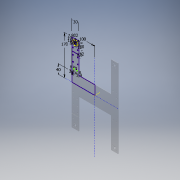
# Autodesk Inventor part: chassis mit motorlöcher
Saved by Autodesk Inventor 2018 (Build 220112000, 112)
## iProperties
Created: 2018-01-20
Part Number: chassis mit motorlöcher
Material: Polycarbonat, rauchfarben
Document SubType Name: Modeling
Designer: fhinstall
Density: 1.2 g/cm^3
Appearance: Polycarbonat - Rauch
Mass: 111.621 g
Surface Area: 687.489 cm^2
Volume: 93.0173 cm^3
Author: fhinstall
Autodesk Inventor part; units mm, degrees
ref_plane "YZ Plane" through (0, 0, 0) normal (1, 0, 0) x (0, 1, 0)
ref_plane "XZ Plane" through (0, 0, 0) normal (0, 1, 0) x (-1, 0, 0)
ref_plane "XY Plane" through (0, 0, 0) normal (0, 0, 1) x (1, 0, 0)
sketch "Skizze1" plane through (0, 0, 0) normal (0, 1, 0) x (-1, 0, 0)
  line L0 (127.3199, 0) -> (-102.7808, 0) construction
  line L1 (0, 142.2638) -> (0, -235.5235) construction
  line L2 (100, 50) -> (100, 0)
  line L3 (70, 40) -> (0, 40)
  line L4 (0, 0) -> (100, 0)
  line L5 (0, 40) -> (0, 0)
  line L6 (100, 50) -> (100, 170)
  line L7 (100, 170) -> (70, 170)
  line L8 (70, 170) -> (70, 40)
  circle A0 centre (95, 36) radius 1.7
  line L9 (100, 140) -> (70, 140) construction
  circle A1 centre (85, 155) radius 4
  circle A2 centre (79.7789, 161.0614) radius 1.7
  circle A3 centre (92.1979, 161.2) radius 1.7
  circle A4 centre (90.2211, 148.9386) radius 1.7
  circle A5 centre (77.8021, 148.8) radius 1.7
  circle A6 centre (85, 155) radius 8 construction
  circle A7 centre (85, 155) radius 9.5 construction
  line L10 (79.7789, 161.0614) -> (90.2211, 148.9386) construction
  line L11 (92.1979, 161.2) -> (77.8021, 148.8) construction
  arc A8 (92.0223, 145.331) -> (96.9015, 153.9244) centre (85, 155) ccw construction
  line L12 (96.9015, 153.9244) -> (96.6242, 153.848) construction
  arc A9 (94.3917, 161.9459) -> (96.6242, 153.848) centre (95.508, 157.8969) ccw construction
  line L13 (94.3917, 161.9459) -> (94.669, 162.0223) construction
  arc A10 (94.669, 162.0223) -> (86.0756, 166.9015) centre (85, 155) ccw construction
  line L14 (86.0756, 166.9015) -> (86.152, 166.6242) construction
  arc A11 (78.0541, 164.3917) -> (86.152, 166.6242) centre (82.1031, 165.508) ccw construction
  line L15 (78.0541, 164.3917) -> (77.9777, 164.669) construction
  arc A12 (77.9777, 164.669) -> (73.0985, 156.0756) centre (85, 155) ccw construction
  line L16 (73.0985, 156.0756) -> (73.3758, 156.152) construction
  arc A13 (75.6083, 148.0541) -> (73.3758, 156.152) centre (74.492, 152.1031) ccw construction
  line L17 (75.6083, 148.0541) -> (75.331, 147.9777) construction
  arc A14 (75.331, 147.9777) -> (83.9244, 143.0985) centre (85, 155) ccw construction
  line L18 (83.9244, 143.0985) -> (83.848, 143.3758) construction
  arc A15 (91.9459, 145.6083) -> (83.848, 143.3758) centre (87.8969, 144.492) ccw construction
  line L19 (91.9459, 145.6083) -> (92.0223, 145.331) construction
  circle A16 centre (85, 155) radius 4 construction
  circle A17 centre (78.0432, 158.95) radius 1.25 construction
  circle A18 centre (89.6906, 163.2613) radius 1.25 construction
  circle A19 centre (91.9568, 151.05) radius 1.25 construction
  circle A20 centre (80.3094, 146.7387) radius 1.25 construction
  line L20 (70, 117.8095) -> (70, 117.3095)
  line L21 (100, 118) -> (70, 118)
  line L22 (70, 118) -> (70, 117.5)
  line L23 (70, 117.5) -> (100, 117.5)
  line L24 (100, 117.5) -> (100, 118)
  circle A21 centre (95.0005, 132.5) radius 1.7
  circle A22 centre (75.0005, 132.5) radius 1.7
  circle A23 centre (75, 105.2) radius 1.7
  circle A24 centre (95, 105.2) radius 1.7
  circle A25 centre (95, 79.2) radius 1.7
  circle A26 centre (75, 79.2) radius 1.7
  circle A27 centre (95.0005, 132.5) radius 1.7
  circle A28 centre (75.0005, 132.5) radius 1.7
  circle A29 centre (75, 105.2) radius 1.7
  circle A30 centre (95, 105.2) radius 1.7
  circle A31 centre (95, 79.2) radius 1.7
  circle A32 centre (75, 79.2) radius 1.7
  circle A33 centre (78, 54.3143) radius 1.7
  circle A34 centre (92, 54.3143) radius 1.7
  dimension "d75" = 19
  dimension "d10" = 100
  dimension "d12" = 30
  dimension "d13" = 170
  dimension "d14" = 40
  dimension "d22" = 5
  dimension "d23" = 4
  dimension "d26" = 3.4
  dimension "d59" = 30
  dimension "d60" = 8
  dimension "d61" = 15
  dimension "d64" = 3.4
  dimension "d65" = 3.4
  dimension "d66" = 3.4
  dimension "d67" = 3.4
  dimension "d70" = 7.8021
  dimension "d74" = 16
  dimension "d76" = 90
  dimension "d78" = 0.5
  dimension "d79" = 52
  dimension "d82" = 3.4
  dimension "d83" = 3.4
  dimension "d84" = 8
  dimension "d85" = 8
  constraints: 34 end point, 21 centre point, 10 coincident, 10 point on line, 7 perpendicular, 6 concentric, 3 midpoint, 2 horizontal, 2 parallel, 2 point on circle, 2 vertical, 1 collinear, 15 other
  measures "d10" distance between parallel lines of L1 L2
  measures "d12" distance of L6.end L7.end
  measures "d13" distance between parallel lines of L0 L7
  measures "d14" distance between parallel lines of L0 L3
  measures "d22" distance from line of L2 A0.centre
  measures "d23" distance from line of L3 A0.centre
  measures "d26" diameter of A0
  measures "d59" distance between parallel lines of L9 L7
  measures "d60" diameter of A1
  measures "d61" distance from line of L9 A1.centre
  measures "d64" diameter of A5
  measures "d65" diameter of A4
  measures "d66" diameter of A3
  measures "d67" diameter of A2
  measures "d70" distance from line of L6 L11.start
  measures "d74" diameter of A6
  measures "d76" angle of L10 L11
  measures "d78" distance of L22.end L21.end
  measures "d79" distance between parallel lines of L7 L21
  measures "d82" diameter of A33
  measures "d83" diameter of A34
  measures "d84" distance from line of L8 A33.centre
  measures "d85" distance from line of L6 A34.centre
extrude "Extrusion1" add sketch "Skizze1" along normal blind 3 contours L2 L4 L5 L3 L8 L23 L6 | L21 L8 L7 L6
ref_plane "Arbeitsebene1" through (0, 0, 40) normal (1, 0, 0) x (0, 1, 0)
ref_plane "Arbeitsebene2" through (0, 3, 0) normal (0, 0, -1) x (-1, 0, 0)
mirror "Spiegeln1" about plane through (0, 3, 0) normal (0, 0, -1) of "Extrusion1"
pattern_circular "Runde Anordnung1" count 2 over 360 about axis through (0, 3, 0) along (0, -1, 0) of "Extrusion1"
mirror "Spiegeln2" about plane through (0, 0, 40) normal (1, 0, 0) of "Extrusion1"
mirror "Spiegeln3" about plane through (0, 3, 0) normal (0, 0, -1) of "Extrusion1"
sketch "Skizze7" plane through (0, 0, 0) normal (0, -1, 0) x (1, 0, 0)
  circle A0 centre (-95, -36) radius 1.7 projected
  circle A1 centre (-75, -105.2) radius 1.7 projected
  circle A2 centre (-95, -105.2) radius 1.7 projected
  circle A3 centre (-95, -79.2) radius 1.7 projected
  circle A4 centre (-75, -79.2) radius 1.7 projected
  line L0 (-70, -40) -> (70, -40) projected
  line L1 (70, -117.5) -> (70, -40) projected
  line L2 (70, -117.5) -> (100, -117.5) projected
  line L3 (100, -117.5) -> (100, 117.5) projected
  line L4 (70, 117.5) -> (100, 117.5) projected
  line L5 (70, 117.5) -> (70, 40) projected
  line L6 (-70, 40) -> (70, 40) projected
  line L7 (-70, 117.5) -> (-70, 40) projected
  line L8 (-70, 117.5) -> (-100, 117.5) projected
  line L9 (-100, 117.5) -> (-100, -117.5) projected
  line L10 (-70, -117.5) -> (-100, -117.5) projected
  line L11 (-70, -117.5) -> (-70, -40) projected
  circle A5 centre (95, 36) radius 1.7 projected
  circle A6 centre (75, 105.2) radius 1.7 projected
  circle A7 centre (95, 105.2) radius 1.7 projected
  circle A8 centre (95, 79.2) radius 1.7 projected
  circle A9 centre (75, 79.2) radius 1.7 projected
  circle A10 centre (95, -36) radius 1.7 projected
  circle A11 centre (75, -105.2) radius 1.7 projected
  circle A12 centre (95, -105.2) radius 1.7 projected
  circle A13 centre (95, -79.2) radius 1.7 projected
  circle A14 centre (75, -79.2) radius 1.7 projected
  circle A15 centre (-75, 79.2) radius 1.7 projected
  circle A16 centre (-95, 79.2) radius 1.7 projected
  circle A17 centre (-95, 105.2) radius 1.7 projected
  circle A18 centre (-75, 105.2) radius 1.7 projected
  circle A19 centre (-95, 36) radius 1.7 projected
  line L12 (100, 118) -> (70, 118) projected
  line L13 (100, 118) -> (100, 170) projected
  line L14 (100, 170) -> (70, 170) projected
  line L15 (70, 170) -> (70, 118) projected
  circle A20 centre (79.7789, 161.0614) radius 1.7 projected
  circle A21 centre (92.1979, 161.2) radius 1.7 projected
  circle A22 centre (90.2211, 148.9386) radius 1.7 projected
  circle A23 centre (77.8021, 148.8) radius 1.7 projected
  circle A24 centre (95.0005, 132.5) radius 1.7 projected
  circle A25 centre (75.0005, 132.5) radius 1.7 projected
  circle A26 centre (85, 155) radius 4 projected
  line L16 (100, -118) -> (70, -118) projected
  line L17 (70, -170) -> (70, -118) projected
  line L18 (100, -170) -> (70, -170) projected
  line L19 (100, -118) -> (100, -170) projected
  circle A27 centre (79.7789, -161.0614) radius 1.7 projected
  circle A28 centre (92.1979, -161.2) radius 1.7 projected
  circle A29 centre (90.2211, -148.9386) radius 1.7 projected
  circle A30 centre (77.8021, -148.8) radius 1.7 projected
  circle A31 centre (95.0005, -132.5) radius 1.7 projected
  circle A32 centre (75.0005, -132.5) radius 1.7 projected
  circle A33 centre (85, -155) radius 4 projected
  line L20 (100, 117.5) -> (70, 117.5) projected
  line L21 (100, 118) -> (100, 170) projected
  line L22 (100, 117.5) -> (100, 118)
  line L23 (70, 118) -> (70, 117.5)
  line L24 (70, -117.5) -> (100, -117.5) projected
  line L25 (70, -117.5) -> (70, -40) projected
  line L26 (70, -117.5) -> (70, -118)
  line L27 (100, -118) -> (100, -170) projected
  line L28 (100, -117.5) -> (100, -118)
  point P0 (0, 0)
  constraints: 8 end point, 3 collinear, 1 vertical
extrude "Extrusion6" add sketch "Skizze7" against normal blind 3 contours L2 L28 L16 L26 | L4 L23 L12 L22 | A6 | A7 | A8 | A9 | A11 | A12 | A13 | A14 | A24 | A25 | A31 | A32
